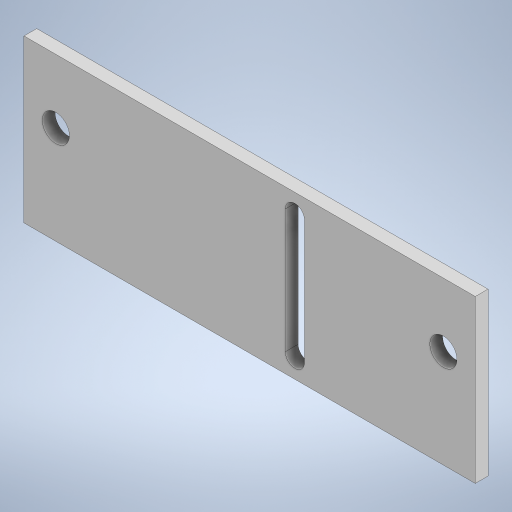
# Autodesk Inventor part: Ultrasonic Sensor 2.0
Saved by Autodesk Inventor 2024 (Build 280153000, 153)
## iProperties
Created: 2023-10-23
Part Number: Ultrasonic Sensor 2.0
Material: Generic
Document SubType Name: Modeling
Designer: olson
Density: 1 g/cm^3
Appearance: Default
Author: olson
Autodesk Inventor part; units mm, degrees
ref_plane "YZ Plane" through (0, 0, 0) normal (1, 0, 0) x (0, 1, 0)
ref_plane "XZ Plane" through (0, 0, 0) normal (0, 1, 0) x (-1, 0, 0)
ref_plane "XY Plane" through (0, 0, 0) normal (0, 0, 1) x (1, 0, 0)
sketch "Sketch1" plane through (0, 0, 0) normal (0, 0, 1) x (1, 0, 0)
  line L0 (0, -6.35) -> (25.4, -6.35)
  line L1 (25.4, -6.35) -> (25.4, -31.75)
  line L2 (25.4, -31.75) -> (-25.4, -31.75)
  line L3 (-25.4, -31.75) -> (-25.4, -6.35)
  line L4 (-25.4, -6.35) -> (0, -6.35)
  point P0 (-6.35, -6.35)
  point P1 (6.35, -6.35)
  dimension "d7" = 25.4
  dimension "d8" = 25.4
  dimension "d9" = 50.8
  constraints: 10 end point, 3 perpendicular, 3 point on line, 1 collinear, 1 horizontal
  measures "d7" distance of L0.start L0.end
  measures "d8" distance of L0.end L1.end
  measures "d9" distance of L1.end L2.end
extrude "Extrusion1" add sketch "Sketch1" along normal blind 2
sketch "Sketch2" plane through (0, 0, 2) normal (0, 0, 1) x (1, 0, 0)
  line L0 (-25.4, -6.35) -> (-25.4, -31.75) projected
  line L1 (-25.4, -31.75) -> (7.1, -31.75)
  line L2 (-25.4, -31.75) -> (25.4, -31.75) projected
  line L3 (7.1, -31.75) -> (7.1, -30.75)
  line L4 (7.1, -30.75) -> (7.1, -28.75)
  circle A0 centre (7.1, -28.75) radius 1.5
  circle A1 centre (7.1, -9.35) radius 1.5
  line L5 (5.6, -9.35) -> (5.6, -28.75)
  line L6 (8.6, -9.35) -> (8.6, -28.75)
  point P0 (0, 0)
  dimension "d10" = 32.5
  dimension "d11" = 1
  dimension "d12" = 2
  dimension "d13" = 3
  dimension "d15" = 3
  constraints: 10 end point, 4 point on circle, 4 tangent, 2 centre point, 2 point on line, 1 coincident, 1 vertical
  measures "d10" distance of L0.end L1.end
  measures "d11" distance of L1.end L3.end
  measures "d12" distance of L3.end L4.end
  measures "d13" diameter of A0
  measures "d15" diameter of A1
extrude "Extrusion2" cut sketch "Sketch2" against normal blind 2.54
sketch "Sketch4" plane through (0, 0, 2) normal (0, 0, 1) x (1, 0, 0)
  line L0 (25.4, -6.35) -> (35.4, -6.35)
  line L1 (35.4, -6.35) -> (35.4, -16.35)
  circle A0 centre (30.4, -16.35) radius 2.125
  line L2 (25.4, -6.35) -> (35.4, -6.35)
  line L3 (35.4, -6.35) -> (35.4, -31.75)
  line L4 (35.4, -31.75) -> (25.4, -31.75)
  line L5 (25.4, -31.75) -> (25.4, -6.35)
  line L6 (25.4, -6.35) -> (-25.4, -6.35) projected
  line L7 (25.4, -6.35) -> (0, -6.35)
  line L8 (0, -6.35) -> (0, -31.75)
  line L9 (-25.4, -6.35) -> (-35.4, -6.35)
  line L10 (-35.4, -6.35) -> (-35.4, -16.35)
  circle A1 centre (-30.4, -16.35) radius 2.125
  line L11 (-25.4, -6.35) -> (-35.4, -6.35)
  line L12 (-35.4, -6.35) -> (-35.4, -31.75)
  line L13 (-35.4, -31.75) -> (-25.4, -31.75)
  line L14 (-25.4, -31.75) -> (-25.4, -6.35)
  point P0 (0, 0)
  dimension "d40" = 10
  dimension "d41" = 10
  dimension "d42" = 4.25
  dimension "d43" = 25.4
  constraints: 28 end point, 6 symmetric about line, 2 centre point, 2 horizontal, 2 parallel, 2 perpendicular, 1 midpoint, 1 vertical, 1 other
  measures "d40" distance of L0.start L0.end
  measures "d41" distance of L0.end L1.end
  measures "d42" diameter of A0
  measures "d43" distance of L2.end L3.end
extrude "Extrusion4" add sketch "Sketch4" against normal blind 2
body "Solid1"
